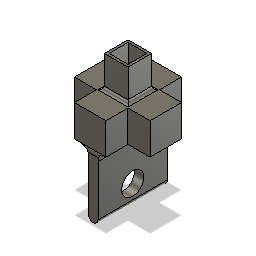
stand for connecting nectary to 80-20 -Single Nectary v2 (Autodesk Fusion 360 design; units mm, degrees)
Autodesk Fusion 360 part; units mm, degrees
sketch "Cross Base 1" plane through (0, 0, 0) normal (1, 0, 0) x (0, 0, -1)
  line L0 (-12, 5) -> (12, 5)
  line L1 (12, 5) -> (12, -5)
  line L2 (12, -5) -> (-12, -5)
  line L3 (-12, -5) -> (-12, 5)
  line L4 (-12, 0) -> (12, 0) construction
  line L5 (0, 5) -> (0, -5) construction
  dimension "d5" = 24
  dimension "d6" = 10
extrude "Extrude3" add sketch "Cross Base 1" along normal mid plane 10
sketch "Cross Base 2" plane through (0, 0, 0) normal (0, 0, 1) x (1, 0, 0)
  line L0 (-12, 5) -> (12, 5)
  line L1 (12, 5) -> (12, -5)
  line L2 (12, -5) -> (-12, -5)
  line L3 (-12, -5) -> (-12, 5)
  line L4 (-12, 0) -> (12, 0) construction
  line L5 (0, 5) -> (0, -5) construction
  dimension "d11" = 24
  dimension "d12" = 10
extrude "Extrude4" add sketch "Cross Base 2" along normal mid plane 10
sketch "Rod to hold nectary" plane through (0, 5, 0) normal (0, 1, 0) x (-1, 0, 0)
  line L0 (5, 5) -> (5, 12)
  line L1 (5, 12) -> (-5, 12)
  line L2 (-5, 12) -> (-5, 5)
  line L3 (-5, 5) -> (-12, 5)
  line L4 (-12, 5) -> (-12, -5)
  line L5 (-12, -5) -> (-5, -5)
  line L6 (-5, -5) -> (-5, -12)
  line L7 (-5, -12) -> (5, -12)
  line L8 (5, -12) -> (5, -5)
  line L9 (5, -5) -> (12, -5)
  line L10 (12, -5) -> (12, 5)
  line L11 (12, 5) -> (5, 5)
  line L12 (0, 0) -> (-0.001, 0) construction
  line L13 (-3.751, 3.75) -> (3.749, 3.75)
  line L14 (3.749, 3.75) -> (3.749, -3.75)
  line L15 (3.749, -3.75) -> (-3.751, -3.75)
  line L16 (-3.751, -3.75) -> (-3.751, 3.75)
  line L17 (-3.751, 3.75) -> (3.749, -3.75) construction
  line L18 (3.749, 3.75) -> (-3.751, -3.75) construction
  dimension "d15" = 0.001
  dimension "d16" = 7.5
  dimension "d42" = 7.5
extrude "Extrude5" add sketch "Rod to hold nectary" along normal blind 10 contours L13 L14 L15 L16
fillet "Fillet1" radius 1 4 edges at (0.001, 5, 3.75) (-3.749, 5, 0) (3.751, 5, 0) (0.001, 5, -3.75)
sketch "hole to hold nectary" plane through (0, 15, 0) normal (0, 1, 0) x (-1, 0, 0)
  line L0 (-3.751, -3.75) -> (3.749, -3.75)
  line L1 (3.749, -3.75) -> (3.749, 3.75)
  line L2 (3.749, 3.75) -> (-3.751, 3.75)
  line L3 (-3.751, 3.75) -> (-3.751, -3.75)
  line L4 (-0.001, -3.75) -> (-0.001, 3.75) construction
  line L5 (-3.751, 0) -> (3.749, 0) construction
  line L6 (-3.001, 3) -> (2.999, 3)
  line L7 (2.999, 3) -> (2.999, -3)
  line L8 (2.999, -3) -> (-3.001, -3)
  line L9 (-3.001, -3) -> (-3.001, 3)
  line L10 (-3.001, 3) -> (2.999, -3) construction
  line L11 (2.999, 3) -> (-3.001, -3) construction
  dimension "d21" = 6
  dimension "d22" = 6
extrude "Extrude6" cut sketch "hole to hold nectary" against normal blind 10 contours L6 L7 L8 L9
sketch "base to aatch tp 80-20" plane through (0, -5, 0) normal (0, -1, 0) x (1, 0, 0)
  line L0 (5, 5) -> (5, 12)
  line L1 (5, 12) -> (-5, 12)
  line L2 (-5, 12) -> (-5, 5)
  line L3 (-5, 5) -> (-12, 5)
  line L4 (-12, 5) -> (-12, -5)
  line L5 (-12, -5) -> (-5, -5)
  line L6 (-5, -5) -> (-5, -12)
  line L7 (-5, -12) -> (5, -12)
  line L8 (5, -12) -> (5, -5)
  line L9 (5, -5) -> (12, -5)
  line L10 (12, -5) -> (12, 5)
  line L11 (12, 5) -> (5, 5)
  line L12 (1.5, -11) -> (-1.5, -11)
  line L13 (-1.5, -11) -> (-1.5, 11)
  line L14 (-1.5, 11) -> (1.5, 11)
  line L15 (1.5, 11) -> (1.5, -11)
  line L16 (1.5, -11) -> (-1.5, 11) construction
  line L17 (-1.5, -11) -> (1.5, 11) construction
  dimension "d27" = 22
  dimension "d28" = 3
extrude "Extrude8" add sketch "base to aatch tp 80-20" along normal blind 21 contours L12 L13 L14 L15
sketch "Sketch7" plane through (1.5, 0, 0) normal (1, 0, 0) x (0, 0, -1)
  line L0 (11, -5) -> (-11, -5)
  line L1 (-11, -5) -> (-11, -26)
  line L2 (-11, -26) -> (11, -26)
  line L3 (11, -26) -> (11, -5)
  line L4 (0, -26) -> (0, -20) construction
  circle A0 centre (0, -20) radius 3.5
  dimension "d35" = 7
  dimension "d38" = 6
  measures "d35" diameter of A0
extrude "Extrude9" cut sketch "Sketch7" against normal up to surface (3 mm away) contours A0
fillet "Fillet2" radius 3.5 4 edges at (0, -5, 11) (-1.5, -5, 0) (1.5, -5, 0) (0, -5, -11)
fillet "Fillet3" radius 1.5 2 edges at (1.5, -26, 0) (-1.5, -26, 0)
